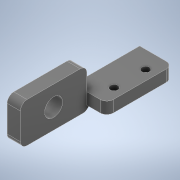
# Autodesk Inventor part: yendstop
Saved by Autodesk Inventor 2022 (Build 260153000, 153)
## iProperties
Created: 2022-07-17
Part Number: yendstop
Material: Genérico
Document SubType Name: Modeling
Designer: JK
Density: 1 g/cm^3
Appearance: Suave - Negro
Author: JK
Autodesk Inventor part; units mm, degrees
ref_plane "YZ Plane" through (0, 0, 0) normal (1, 0, 0) x (0, 1, 0)
ref_plane "XZ Plane" through (0, 0, 0) normal (0, 1, 0) x (-1, 0, 0)
ref_plane "XY Plane" through (0, 0, 0) normal (0, 0, 1) x (1, 0, 0)
sketch "Boceto1" plane through (0, 0, 0) normal (0, 1, 0) x (-1, 0, 0)
  line L0 (8.3442, 9.5108) -> (-1.6558, 9.5108)
  line L1 (-1.6558, 9.5108) -> (-1.6558, -10.3892)
  line L2 (-1.6558, -10.3892) -> (8.3442, -10.3892)
  line L3 (8.3442, -10.3892) -> (8.3442, 9.5108)
  circle A0 centre (1.3442, 4.3108) radius 1.15
  circle A1 centre (1.3442, -5.1892) radius 1.15
  point P0 (0, 0)
  dimension "d0" = 2.3
  dimension "d1" = 9.5
  dimension "d2" = 5.2
  dimension "d3" = 5.2
  dimension "d4" = 3
  dimension "d5" = 7
  constraints: 8 end point, 2 centre point, 2 parallel, 1 equal radius, 1 horizontal, 1 perpendicular
  measures "d0" diameter of A0
  measures "d1" distance of A1.centre A0.centre
  measures "d2" distance from line of L0 A0.centre
  measures "d3" distance from line of L2 A1.centre
  measures "d4" distance from line of A1.centre L1
  measures "d5" distance from line of L3 A0.centre
extrude "Extrusión1" add sketch "Boceto1" against normal blind 3.5
sketch "Boceto2" plane through (-8.3442, 0, -10.3892) normal (-1, 0, 0) x (0, 0, 1)
  line L0 (19.9, 0) -> (0, 0) projected
  line L1 (19.9, 0) -> (39.9, 0)
  line L2 (39.9, 0) -> (39.9, -5)
  line L3 (39.9, -5) -> (19.9, -5)
  line L4 (19.9, -5) -> (19.9, 0)
  line L5 (39.9, 0) -> (19.9, 0)
  line L6 (19.9, 0) -> (19.9, 7)
  line L7 (19.9, 7) -> (39.9, 7)
  line L8 (39.9, 7) -> (39.9, 0)
  circle A0 centre (29.9, 1) radius 2.7
  point P0 (10.3892, 0)
  dimension "d8" = 20
  dimension "d9" = 1
  dimension "d10" = 5.4
  dimension "d11" = 10
  dimension "d12" = 6
  dimension "d13" = 6
  constraints: 16 end point, 4 parallel, 2 horizontal, 2 perpendicular, 1 centre point, 1 collinear
  measures "d8" distance between parallel lines of L4 L2
  measures "d9" distance from line of L0 A0.centre
  measures "d10" diameter of A0
  measures "d11" distance from line of L4 A0.centre
  measures "d12" distance from line of A0.centre L7
  measures "d13" distance from line of L3 A0.centre
extrude "Extrusión2" add sketch "Boceto2" against normal blind 4 contours L6 L7 L8 L1 A0 | L1 A0 L2 L3 L4
fillet "Empalme1" radius 2 7 edges at (-6.3442, -3.5, 9.5108) (-6.3442, -5, 9.5108) (-6.3442, -5, 29.5108) (-6.3442, 7, 29.5108) (-6.3442, 7, 9.5108) (1.6558, -1.75, 9.5108) (1.6558, -1.75, -10.3892)
sketch "Boceto3" plane through (0, -3.5, 0) normal (0, -1, 0) x (1, 0, 0)
  circle A0 centre (-1.3442, 4.3108) radius 1.15 projected
  circle A1 centre (-1.3442, 4.3108) radius 2.15
  circle A2 centre (-1.3442, -5.1892) radius 1.15 projected
  circle A3 centre (-1.3442, -5.1892) radius 2.15
  line L0 (1.1384, 4.3108) -> (-0.1029, 2.1608)
  line L1 (-0.1029, 2.1608) -> (-2.5855, 2.1608)
  line L2 (-2.5855, 2.1608) -> (-3.8268, 4.3108)
  line L3 (-3.8268, 4.3108) -> (-2.5855, 6.4608)
  line L4 (-2.5855, 6.4608) -> (-0.1029, 6.4608)
  line L5 (-0.1029, 6.4608) -> (1.1384, 4.3108)
  line L6 (-3.8268, -5.1892) -> (-2.5855, -3.0392)
  line L7 (-2.5855, -3.0392) -> (-0.1029, -3.0392)
  line L8 (-0.1029, -3.0392) -> (1.1384, -5.1892)
  line L9 (1.1384, -5.1892) -> (-0.1029, -7.3392)
  line L10 (-0.1029, -7.3392) -> (-2.5855, -7.3392)
  line L11 (-2.5855, -7.3392) -> (-3.8268, -5.1892)
  point P0 (0, 0)
  dimension "d17" = 4.3
  constraints: 24 end point, 4 coincident, 2 centre point, 2 horizontal alignment, 2 tangent, 1 equal radius, 26 other
  measures "d17" diameter of A1
extrude "Extrusión3" cut sketch "Boceto3" against normal blind 2 contours A0 | A1 | A1 L5 L0 | A1 L4 L5 | L0 L1 A1 | A1 L3 L4 | L1 L2 A1 | A1 L2 L3 | A2 | A3 | A3 L8 L9 | A3 L7 L8 | L9 L10 A3 | A3 L6 L7 | L10 L11 A3 | A3 L11 L6
